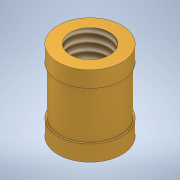
# Autodesk Inventor part: M3_5mm_Insert
Saved by Autodesk Inventor 2020 (Build 240168000, 168)
## iProperties
Created: 2019-12-01
Part Number: M3_5mm_Insert
Material: Generic
Document SubType Name: Modeling
Designer: kylew
Density: 1 g/cm^3
Appearance: Default
Author: kylew
Autodesk Inventor part; units mm, degrees
ref_plane "YZ Plane" through (0, 0, 0) normal (1, 0, 0) x (0, 1, 0)
ref_plane "XZ Plane" through (0, 0, 0) normal (0, 1, 0) x (-1, 0, 0)
ref_plane "XY Plane" through (0, 0, 0) normal (0, 0, 1) x (1, 0, 0)
sketch "Sketch1" plane through (0, 0, 0) normal (1, 0, 0) x (0, 1, 0)
  line L0 (0, 0) -> (0, 2)
  line L1 (0, 0) -> (2, 0) construction
  line L2 (0, 2) -> (-1, 2)
  line L3 (-1, 2) -> (-1, 1.9)
  line L4 (-1, 1.9) -> (-4, 1.9)
  line L5 (-4, 1.9) -> (-4, 2)
  line L6 (-4, 2) -> (-5, 2)
  line L7 (-5, 2) -> (-5, 0)
  line L8 (0, 0) -> (-5, 0)
  line L9 (-6.4, 0) -> (3.4, 0) projected
  dimension "d0" = 2
  dimension "d1" = 90
  dimension "d2" = 1
  dimension "d3" = 0.1
  dimension "d4" = 3
  dimension "d5" = 90
  dimension "d6" = 0.1
  dimension "d7" = 1
  dimension "d8" = 90
  dimension "d9" = 2
  dimension "d10" = 90
  constraints: 18 end point, 6 perpendicular, 2 vertical, 1 horizontal
  measures "d0" distance of L0.start L0.end
  measures "d1" angle of L1 L0
  measures "d2" distance of L0.end L2.end
  measures "d3" distance of L2.end L3.end
  measures "d4" distance of L3.end L4.end
  measures "d5" angle of L3 L4
  measures "d6" distance of L4.end L5.end
  measures "d7" distance of L5.end L6.end
  measures "d8" angle of L6 L5
  measures "d9" distance of L6.end L7.end
  measures "d10" angle of L7 L6
revolve "Revolution1" add sketch "Sketch1" angle 360 about axis through (0, -10, 0) along (0, 1, 0)
sketch "Sketch2" plane through (0, 0, 0) normal (0, 1, 0) x (1, 0, 0)
  point P0 (0, 0)
  point P1 (-0.0069, 0.0128)
hole "Hole1" at (-0.0069, 0, -0.0128) direction (0, -1, 0) diameter 2.459 end through all thread size "M3x0.5" class "6H" standard "ANSI Metric M Profile"
body "Solid1"
